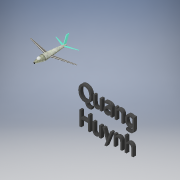
# Autodesk Inventor part: wingi boi0
Saved by Autodesk Inventor 2017 (Build 210142000, 142)
## iProperties
Created: 2019-04-23
Part Number: wingi boi0
Material: Generic
Document SubType Name: Modeling
Designer: qthuynh
Density: 1 g/cm^3
Appearance: Default
Author: qthuynh
Autodesk Inventor part; units mm, degrees
ref_plane "XZ Plane" through (0, 0, 0) normal (0, 1, 0) x (-1, 0, 0)
sketch "Sketch1" plane through (0, 0, 0) normal (0, 0, 1) x (1, 0, 0)
  circle A0 centre (0, 0) radius 25.4
  dimension "d0" = 50.8
  constraints: 1 centre point, 1 coincident
  measures "d0" diameter of A0
extrude "Extrusion1" add sketch "Sketch1" against normal blind 203.2 draft -5
sketch "Sketch2" plane through (0, 0, 0) normal (0, 0, 1) x (1, 0, 0)
  circle A0 centre (0, 0) radius 25.4
  constraints: 1 centre point, 1 coincident
extrude "Extrusion2" add sketch "Sketch2" along normal blind 76.2 draft -13
ref_plane "Work Plane1" through (0, 0, 0) normal (1, 0, 0) x (0, 1, 0)
ref_plane "Work Plane2" through (203.2, 0, 0) normal (1, 0, 0) x (0, 1, 0)
sketch "Sketch4" plane through (0, 0, 0) normal (1, 0, 0) x (0, 1, 0)
  ellipse E0 centre (0, -44.6525) end of major axis (0, -61.2958) minor radius 3.5254
  point P0 (0, 0)
  constraints: 2 other
sketch "Sketch5" plane through (203.2, 0, 0) normal (1, 0, 0) x (0, 1, 0)
  ellipse E0 centre (0, -94.3799) end of major axis (0, -99.7321) minor radius 1.468
  point P0 (0, 0)
  constraints: 2 other
loft "Loft1" add profiles "Sketch5", "Sketch4"
ref_plane "Work Plane3" through (101.6, 0, 0) normal (1, 0, 0) x (0, 1, 0)
sketch "Sketch7" plane through (101.6, 0, 0) normal (1, 0, 0) x (0, 1, 0)
  ellipse E0 centre (0, -215.8771) end of major axis (0, -217.8432) minor radius 1.6297
  point P0 (0, 0)
  constraints: 2 other
sketch "Sketch10" plane through (0, 0, 0) normal (1, 0, 0) x (0, 1, 0)
  ellipse E0 centre (0, -181.8764) end of major axis (0, -190.9103) minor radius 1.7763
  point P0 (0, 0)
  constraints: 2 other
loft "Loft2" add profiles "Sketch7", "Sketch10"
ref_plane "Work Plane4" through (0, 0, -125.4125) normal (0, 0, 1) x (1, 0, 0)
ref_plane "Work Plane5" through (0, 0, 87.3125) normal (0, 0, 1) x (1, 0, 0)
sketch "Sketch14" plane through (0, 0, 87.3125) normal (0, 0, 1) x (1, 0, 0)
  line L0 (419.757, 90.143) -> (690.1861, 90.143) construction
  line L1 (690.1861, 90.143) -> (690.1861, 10.0159) construction
  line L2 (690.1861, 10.0159) -> (419.757, 10.0159) construction
  line L3 (419.757, 10.0159) -> (419.757, 90.143) construction
  spline S0 degree 2 poles (538.1119, -70.6139) (533.4806, -71.7459) (523.3947, -72.981) (518.3518, -72.981) knots 0 0 0 1 2 2 2
  spline S1 degree 2 poles (518.3518, -72.981) (504.0463, -72.981) (486.2416, -57.0288) (485.4182, -42.2087) knots 0 0 0 1 2 2 2
  spline S2 degree 2 poles (485.4182, -42.2087) (484.2861, -42.2087) (482.3307, -42.2087) (481.5074, -42.2087) knots 0 0 0 1 2 2 2
  spline S3 degree 2 poles (481.5074, -42.2087) (468.6427, -42.2087) (447.9563, -33.4607) (440.5463, -24.9186) knots 0 0 0 1 2 2 2
  spline S4 degree 2 poles (440.5463, -24.9186) (433.2391, -16.4793) (425.4174, 8.2208) (425.4174, 23.8643) knots 0 0 0 1 2 2 2
  spline S5 degree 2 poles (425.4174, 23.8643) (425.4174, 39.9194) (433.342, 64.2079) (440.6492, 72.8529) knots 0 0 0 1 2 2 2
  spline S6 degree 2 poles (440.6492, 72.8529) (448.0592, 81.3951) (468.7456, 90.143) (481.5074, 90.143) knots 0 0 0 1 2 2 2
  spline S7 degree 2 poles (481.5074, 90.143) (494.4749, 90.143) (515.2643, 81.0863) (522.4685, 72.8529) knots 0 0 0 1 2 2 2
  spline S8 degree 2 poles (522.4685, 72.8529) (529.6727, 64.5166) (537.7002, 39.7135) (537.7002, 23.8643) knots 0 0 0 1 2 2 2
  spline S9 degree 2 poles (537.7002, 23.8643) (537.7002, -0.8359) (518.4547, -32.9461) (501.6792, -38.6066) knots 0 0 0 1 2 2 2
  spline S10 degree 2 poles (501.6792, -38.6066) (502.0908, -43.3408) (504.5608, -50.9566) (506.5163, -53.1179) knots 0 0 0 1 2 2 2
  spline S11 degree 2 poles (506.5163, -53.1179) (508.8834, -55.7938) (515.3672, -58.2638) (521.1305, -58.2638) knots 0 0 0 1 2 2 2
  spline S12 degree 2 poles (521.1305, -58.2638) (524.5268, -58.2638) (533.7894, -56.1025) (535.8477, -55.2792) knots 0 0 0 1 2 2 2
  line L4 (535.8477, -55.2792) -> (538.1119, -55.2792)
  line L5 (538.1119, -55.2792) -> (538.1119, -70.6139)
  spline S13 degree 2 poles (520.1014, 23.8643) (520.1014, 36.5231) (514.6467, 55.9745) (509.7067, 62.3554) knots 0 0 0 1 2 2 2
  spline S14 degree 2 poles (509.7067, 62.3554) (504.6638, 68.9421) (490.4612, 75.5288) (481.6103, 75.5288) knots 0 0 0 1 2 2 2
  spline S15 degree 2 poles (481.6103, 75.5288) (472.4506, 75.5288) (458.6597, 69.1479) (453.4109, 62.3554) knots 0 0 0 1 2 2 2
  spline S16 degree 2 poles (453.4109, 62.3554) (448.368, 55.8716) (443.0163, 36.2143) (443.0163, 23.8643) knots 0 0 0 1 2 2 2
  spline S17 degree 2 poles (443.0163, 23.8643) (443.0163, -1.1446) (464.0114, -27.8002) (481.6103, -27.8002) knots 0 0 0 1 2 2 2
  spline S18 degree 2 poles (481.6103, -27.8002) (499.2091, -27.8002) (520.1014, -1.1446) (520.1014, 23.8643) knots 0 0 0 1 2 2 2
  line L6 (629.0908, -39.5328) -> (613.0357, -39.5328)
  line L7 (613.0357, -39.5328) -> (613.0357, -29.0352)
  spline S19 degree 2 poles (613.0357, -29.0352) (605.6257, -35.519) (592.3493, -42.2087) (584.116, -42.2087) knots 0 0 0 1 2 2 2
  spline S20 degree 2 poles (584.116, -42.2087) (577.9409, -42.2087) (566.9288, -38.092) (562.915, -33.6665) knots 0 0 0 1 2 2 2
  spline S21 degree 2 poles (562.915, -33.6665) (558.7983, -29.2411) (554.2699, -15.7589) (554.2699, -6.0847) knots 0 0 0 1 2 2 2
  line L8 (554.2699, -6.0847) -> (554.2699, 55.7686)
  line L9 (554.2699, 55.7686) -> (570.325, 55.7686)
  line L10 (570.325, 55.7686) -> (570.325, 1.4283)
  spline S22 degree 2 poles (570.325, 1.4283) (570.325, -6.1876) (571.4571, -16.1706) (573.4125, -19.8756) knots 0 0 0 1 2 2 2
  spline S23 degree 2 poles (573.4125, -19.8756) (575.368, -23.5806) (582.0576, -26.9769) (588.3356, -26.9769) knots 0 0 0 1 2 2 2
  spline S24 degree 2 poles (588.3356, -26.9769) (594.2019, -26.9769) (607.4782, -20.2873) (613.0357, -15.4502) knots 0 0 0 1 2 2 2
  line L11 (613.0357, -15.4502) -> (613.0357, 55.7686)
  line L12 (613.0357, 55.7686) -> (629.0908, 55.7686)
  line L13 (629.0908, 55.7686) -> (629.0908, -39.5328)
  spline S25 degree 2 poles (705.4555, -29.4469) (703.5001, -30.8878) (696.9134, -36.0336) (693.8258, -37.5774) knots 0 0 0 1 2 2 2
  spline S26 degree 2 poles (693.8258, -37.5774) (689.6062, -39.8416) (681.6816, -42.2087) (674.4774, -42.2087) knots 0 0 0 1 2 2 2
  spline S27 degree 2 poles (674.4774, -42.2087) (668.6111, -42.2087) (658.0106, -37.7832) (653.9968, -33.7694) knots 0 0 0 1 2 2 2
  spline S28 degree 2 poles (653.9968, -33.7694) (650.1889, -29.8586) (645.5576, -18.3318) (645.5576, -11.951) knots 0 0 0 1 2 2 2
  spline S29 degree 2 poles (645.5576, -11.951) (645.5576, -2.0709) (653.8939, 11.9259) (662.9506, 15.9396) knots 0 0 0 1 2 2 2
  spline S30 degree 2 poles (662.9506, 15.9396) (670.9782, 19.6447) (692.7967, 22.4234) (705.4555, 23.1438) knots 0 0 0 1 2 2 2
  line L14 (705.4555, 23.1438) -> (705.4555, 26.2314)
  spline S31 degree 2 poles (705.4555, 26.2314) (705.4555, 31.7889) (702.0592, 38.6844) (698.9717, 40.6398) knots 0 0 0 1 2 2 2
  spline S32 degree 2 poles (698.9717, 40.6398) (695.8842, 42.5952) (687.0333, 43.8302) (682.2991, 43.8302) knots 0 0 0 1 2 2 2
  spline S33 degree 2 poles (682.2991, 43.8302) (676.7416, 43.8302) (661.7156, 40.5369) (654.2027, 37.3464) knots 0 0 0 1 2 2 2
  line L15 (654.2027, 37.3464) -> (653.2764, 37.3464)
  line L16 (653.2764, 37.3464) -> (653.2764, 53.7103)
  spline S34 degree 2 poles (653.2764, 53.7103) (657.7018, 54.9453) (674.2715, 58.0328) (682.402, 58.0328) knots 0 0 0 1 2 2 2
  spline S35 degree 2 poles (682.402, 58.0328) (692.2821, 58.0328) (705.7642, 54.9453) (711.1159, 50.9315) knots 0 0 0 1 2 2 2
  spline S36 degree 2 poles (711.1159, 50.9315) (716.3647, 47.0207) (721.5106, 34.5677) (721.5106, 25.6139) knots 0 0 0 1 2 2 2
  line L17 (721.5106, 25.6139) -> (721.5106, -39.5328)
  line L18 (721.5106, -39.5328) -> (705.4555, -39.5328)
  line L19 (705.4555, -39.5328) -> (705.4555, -29.4469)
  line L20 (705.4555, -16.0677) -> (705.4555, 10.3821)
  spline S37 degree 2 poles (705.4555, 10.3821) (699.6921, 9.8675) (682.2991, 8.1179) (676.8445, 6.4712) knots 0 0 0 1 2 2 2
  spline S38 degree 2 poles (676.8445, 6.4712) (670.4636, 4.5158) (662.1273, -3.6147) (662.1273, -10.8189) knots 0 0 0 1 2 2 2
  spline S39 degree 2 poles (662.1273, -10.8189) (662.1273, -19.0523) (671.3899, -27.3886) (680.2407, -27.3886) knots 0 0 0 1 2 2 2
  spline S40 degree 2 poles (680.2407, -27.3886) (687.7537, -27.3886) (700.1038, -20.9048) (705.4555, -16.0677) knots 0 0 0 1 2 2 2
  line L21 (818.8704, -39.5328) -> (802.8153, -39.5328)
  line L22 (802.8153, -39.5328) -> (802.8153, 14.8075)
  spline S41 degree 2 poles (802.8153, 14.8075) (802.8153, 21.3942) (801.5803, 32.7152) (799.7278, 36.1114) knots 0 0 0 1 2 2 2
  spline S42 degree 2 poles (799.7278, 36.1114) (797.7724, 39.7135) (790.774, 43.2127) (784.8048, 43.2127) knots 0 0 0 1 2 2 2
  spline S43 degree 2 poles (784.8048, 43.2127) (778.8356, 43.2127) (766.1767, 36.8318) (760.1046, 31.686) knots 0 0 0 1 2 2 2
  line L23 (760.1046, 31.686) -> (760.1046, -39.5328)
  line L24 (760.1046, -39.5328) -> (744.0495, -39.5328)
  line L25 (744.0495, -39.5328) -> (744.0495, 55.7686)
  line L26 (744.0495, 55.7686) -> (760.1046, 55.7686)
  line L27 (760.1046, 55.7686) -> (760.1046, 45.1682)
  spline S44 degree 2 poles (760.1046, 45.1682) (767.3088, 51.6519) (781.2027, 58.4445) (789.0244, 58.4445) knots 0 0 0 1 2 2 2
  spline S45 degree 2 poles (789.0244, 58.4445) (803.0211, 58.4445) (818.8704, 39.9194) (818.8704, 22.3205) knots 0 0 0 1 2 2 2
  line L28 (818.8704, 22.3205) -> (818.8704, -39.5328)
  spline S46 degree 2 poles (844.8056, -54.7646) (846.4523, -55.485) (852.7302, -57.7492) (856.744, -58.6754) knots 0 0 0 1 2 2 2
  spline S47 degree 2 poles (856.744, -58.6754) (861.1694, -59.8075) (868.6824, -61.1455) (873.1078, -61.1455) knots 0 0 0 1 2 2 2
  spline S48 degree 2 poles (873.1078, -61.1455) (880.5179, -61.1455) (890.8096, -57.2346) (893.6913, -53.7354) knots 0 0 0 1 2 2 2
  spline S49 degree 2 poles (893.6913, -53.7354) (896.4701, -50.2362) (898.6313, -41.0766) (898.6313, -35.2103) knots 0 0 0 1 2 2 2
  line L29 (898.6313, -35.2103) -> (898.6313, -26.874)
  spline S50 degree 2 poles (898.6313, -26.874) (892.1476, -32.5344) (879.6946, -37.8861) (870.3291, -37.8861) knots 0 0 0 1 2 2 2
  spline S51 degree 2 poles (870.3291, -37.8861) (854.0681, -37.8861) (834.8226, -13.7006) (834.8226, 9.0442) knots 0 0 0 1 2 2 2
  spline S52 degree 2 poles (834.8226, 9.0442) (834.8226, 20.8797) (841.5122, 39.1989) (847.0698, 45.6827) knots 0 0 0 1 2 2 2
  spline S53 degree 2 poles (847.0698, 45.6827) (852.4215, 51.7549) (867.1386, 58.4445) (874.9604, 58.4445) knots 0 0 0 1 2 2 2
  spline S54 degree 2 poles (874.9604, 58.4445) (882.3704, 58.4445) (893.1767, 54.9453) (898.6313, 51.7549) knots 0 0 0 1 2 2 2
  line L30 (898.6313, 51.7549) -> (899.5576, 55.7686)
  line L31 (899.5576, 55.7686) -> (914.6864, 55.7686)
  line L32 (914.6864, 55.7686) -> (914.6864, -28.6236)
  spline S55 degree 2 poles (914.6864, -28.6236) (914.6864, -52.9121) (893.5884, -75.5539) (871.8728, -75.5539) knots 0 0 0 1 2 2 2
  spline S56 degree 2 poles (871.8728, -75.5539) (864.8745, -75.5539) (850.2602, -73.2897) (843.9822, -71.4372) knots 0 0 0 1 2 2 2
  line L33 (843.9822, -71.4372) -> (843.9822, -54.7646)
  line L34 (843.9822, -54.7646) -> (844.8056, -54.7646)
  line L35 (898.6313, -13.7006) -> (898.6313, 38.6844)
  spline S57 degree 2 poles (898.6313, 38.6844) (892.6621, 41.566) (882.5762, 44.0361) (877.5333, 44.0361) knots 0 0 0 1 2 2 2
  spline S58 degree 2 poles (877.5333, 44.0361) (865.389, 44.0361) (851.3923, 26.1284) (851.3923, 9.3529) knots 0 0 0 1 2 2 2
  spline S59 degree 2 poles (851.3923, 9.3529) (851.3923, -6.4964) (861.9928, -23.066) (873.9312, -23.066) knots 0 0 0 1 2 2 2
  spline S60 degree 2 poles (873.9312, -23.066) (880.2091, -23.066) (893.3826, -18.126) (898.6313, -13.7006) knots 0 0 0 1 2 2 2
  line L36 (524.8356, -248.635) -> (507.9571, -248.635)
  line L37 (507.9571, -248.635) -> (507.9571, -186.4729)
  line L38 (507.9571, -186.4729) -> (449.5001, -186.4729)
  line L39 (449.5001, -186.4729) -> (449.5001, -248.635)
  line L40 (449.5001, -248.635) -> (432.6216, -248.635)
  line L41 (432.6216, -248.635) -> (432.6216, -121.635)
  line L42 (432.6216, -121.635) -> (449.5001, -121.635)
  line L43 (449.5001, -121.635) -> (449.5001, -171.447)
  line L44 (449.5001, -171.447) -> (507.9571, -171.447)
  line L45 (507.9571, -171.447) -> (507.9571, -121.635)
  line L46 (507.9571, -121.635) -> (524.8356, -121.635)
  line L47 (524.8356, -121.635) -> (524.8356, -248.635)
  line L48 (623.4304, -248.635) -> (607.3753, -248.635)
  line L49 (607.3753, -248.635) -> (607.3753, -238.1374)
  spline S61 degree 2 poles (607.3753, -238.1374) (599.9652, -244.6212) (586.6889, -251.3108) (578.4555, -251.3108) knots 0 0 0 1 2 2 2
  spline S62 degree 2 poles (578.4555, -251.3108) (572.2805, -251.3108) (561.2683, -247.1941) (557.2545, -242.7687) knots 0 0 0 1 2 2 2
  spline S63 degree 2 poles (557.2545, -242.7687) (553.1378, -238.3432) (548.6095, -224.8611) (548.6095, -215.1868) knots 0 0 0 1 2 2 2
  line L50 (548.6095, -215.1868) -> (548.6095, -153.3335)
  line L51 (548.6095, -153.3335) -> (564.6646, -153.3335)
  line L52 (564.6646, -153.3335) -> (564.6646, -207.6739)
  spline S64 degree 2 poles (564.6646, -207.6739) (564.6646, -215.2898) (565.7967, -225.2727) (567.7521, -228.9778) knots 0 0 0 1 2 2 2
  spline S65 degree 2 poles (567.7521, -228.9778) (569.7075, -232.6828) (576.3972, -236.0791) (582.6751, -236.0791) knots 0 0 0 1 2 2 2
  spline S66 degree 2 poles (582.6751, -236.0791) (588.5414, -236.0791) (601.8177, -229.3894) (607.3753, -224.5523) knots 0 0 0 1 2 2 2
  line L53 (607.3753, -224.5523) -> (607.3753, -153.3335)
  line L54 (607.3753, -153.3335) -> (623.4304, -153.3335)
  line L55 (623.4304, -153.3335) -> (623.4304, -248.635)
  line L56 (721.5106, -153.3335) -> (670.2578, -283.7298)
  line L57 (670.2578, -283.7298) -> (653.0706, -283.7298)
  line L58 (653.0706, -283.7298) -> (670.1548, -244.0037)
  line L59 (670.1548, -244.0037) -> (635.5746, -153.3335)
  line L60 (635.5746, -153.3335) -> (652.8647, -153.3335)
  line L61 (652.8647, -153.3335) -> (678.9028, -223.9348)
  line L62 (678.9028, -223.9348) -> (704.838, -153.3335)
  line L63 (704.838, -153.3335) -> (721.5106, -153.3335)
  line L64 (808.4758, -248.635) -> (792.4206, -248.635)
  line L65 (792.4206, -248.635) -> (792.4206, -194.2946)
  spline S67 degree 2 poles (792.4206, -194.2946) (792.4206, -187.7079) (791.1856, -176.387) (789.3331, -172.9907) knots 0 0 0 1 2 2 2
  spline S68 degree 2 poles (789.3331, -172.9907) (787.3777, -169.3886) (780.3793, -165.8894) (774.4101, -165.8894) knots 0 0 0 1 2 2 2
  spline S69 degree 2 poles (774.4101, -165.8894) (768.4409, -165.8894) (755.7821, -172.2703) (749.71, -177.4162) knots 0 0 0 1 2 2 2
  line L66 (749.71, -177.4162) -> (749.71, -248.635)
  line L67 (749.71, -248.635) -> (733.6548, -248.635)
  line L68 (733.6548, -248.635) -> (733.6548, -153.3335)
  line L69 (733.6548, -153.3335) -> (749.71, -153.3335)
  line L70 (749.71, -153.3335) -> (749.71, -163.934)
  spline S70 degree 2 poles (749.71, -163.934) (756.9142, -157.4502) (770.808, -150.6577) (778.6297, -150.6577) knots 0 0 0 1 2 2 2
  spline S71 degree 2 poles (778.6297, -150.6577) (792.6265, -150.6577) (808.4758, -169.1828) (808.4758, -186.7816) knots 0 0 0 1 2 2 2
  line L71 (808.4758, -186.7816) -> (808.4758, -248.635)
  line L72 (905.8356, -248.635) -> (889.7805, -248.635)
  line L73 (889.7805, -248.635) -> (889.7805, -194.2946)
  spline S72 degree 2 poles (889.7805, -194.2946) (889.7805, -187.7079) (888.5454, -176.387) (886.6929, -172.9907) knots 0 0 0 1 2 2 2
  spline S73 degree 2 poles (886.6929, -172.9907) (884.7375, -169.3886) (877.7391, -165.8894) (871.7699, -165.8894) knots 0 0 0 1 2 2 2
  spline S74 degree 2 poles (871.7699, -165.8894) (865.8007, -165.8894) (853.1419, -172.2703) (847.0698, -177.4162) knots 0 0 0 1 2 2 2
  line L74 (847.0698, -177.4162) -> (847.0698, -248.635)
  line L75 (847.0698, -248.635) -> (831.0147, -248.635)
  line L76 (831.0147, -248.635) -> (831.0147, -115.9745)
  line L77 (831.0147, -115.9745) -> (847.0698, -115.9745)
  line L78 (847.0698, -115.9745) -> (847.0698, -163.934)
  spline S75 degree 2 poles (847.0698, -163.934) (854.274, -157.4502) (868.1678, -150.6577) (875.9895, -150.6577) knots 0 0 0 1 2 2 2
  spline S76 degree 2 poles (875.9895, -150.6577) (889.9863, -150.6577) (905.8356, -169.1828) (905.8356, -186.7816) knots 0 0 0 1 2 2 2
  line L79 (905.8356, -186.7816) -> (905.8356, -248.635)
  point P0 (0, 0)
  constraints: 2 other
extrude "Extrusion5" add sketch "Sketch14" along normal blind 25.4
sketch "Sketch15" plane through (0, 0, 0) normal (1, 0, 0) x (0, 1, 0)
  arc A0 (17.0408, 23.3182) -> (10.3735, 50.8208) centre (12.0406, 36.6655) ccw
  line L0 (10.3735, 50.8208) -> (17.0408, 23.3182)
  point P0 (0, 0)
  constraints: 2 end point, 2 point on circle, 1 centre point
revolve "Revolution1" add sketch "Sketch15" angle 360 about axis through (0, 10.3735, 50.8208) along (0, 0.2356, -0.9718501)
mirror "Mirror1" about plane through (0, 0, 0) normal (1, 0, 0) of "Loft1"
mirror "Mirror2" about plane through (0, 0, 0) normal (1, 0, 0) of "Loft2"
sketch "Sketch19" plane through (0, 0, 0) normal (1, 0, 0) x (0, 1, 0)
  line L0 (0, -176.7064) -> (72.172, -206.1015)
  line L1 (72.172, -206.1015) -> (72.172, -229.6288)
  line L2 (72.172, -229.6288) -> (0, -200.2337)
  line L3 (0, -176.7064) -> (0, -200.2337)
  line L4 (0, -217.8432) -> (0, -193.1636) projected
  line L5 (72.172, -229.6288) -> (72.172, -206.1015)
  point P0 (0, 0)
  constraints: 10 end point, 2 collinear, 1 parallel, 1 vertical
extrude "Extrusion6" add sketch "Sketch19" along normal mid plane 5.1435
body "Solid1"
